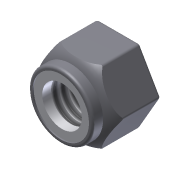
# Autodesk Inventor part: 10-32 regular lock nut
Saved by Autodesk Inventor 2011 (Build 150239000, 239)
## iProperties
Created: 2011-07-10
Part Number: 10-32 regular lock nut
Document SubType Name: Modeling
Designer: Dan Niemitalo
Density: 6.53812 g/cm^3
Material: Steel
Mass: 8.618 g
Surface Area: 11.454 cm^2
Volume: 1.31812 cm^3
Author: Dan Niemitalo
Autodesk Inventor part; units mm, degrees
ref_plane "YZ Plane" through (0, 0, 0) normal (1, 0, 0) x (0, 1, 0)
ref_plane "XZ Plane" through (0, 0, 0) normal (0, 1, 0) x (-1, 0, 0)
ref_plane "XY Plane" through (0, 0, 0) normal (0, 0, 1) x (1, 0, 0)
sketch "Sketch1" plane through (0, 0, 0) normal (0, 0, 1) x (1, 0, 0)
  line L0 (-4.1244, 7.1437) -> (4.1244, 7.1437)
  line L1 (4.1244, 7.1437) -> (8.2489, 0)
  line L2 (8.2489, 0) -> (4.1244, -7.1437)
  line L3 (4.1244, -7.1437) -> (-4.1244, -7.1437)
  line L4 (-4.1244, -7.1437) -> (-8.2489, 0)
  line L5 (-8.2489, 0) -> (-4.1244, 7.1437)
  point P0 (0, 0)
  point P1 (0, 0)
  dimension "d0" = 14.2875
  constraints: 12 end point, 1 coincident, 1 horizontal, 13 other
  measures "d0" distance between parallel lines of L3 L0
extrude "Extrusion1" add sketch "Sketch1" along normal blind 9.525
sketch "Sketch3" plane through (0, 0, 9.525) normal (0, 0, 1) x (1, 0, 0)
  circle A0 centre (0, 0) radius 6.35
  dimension "d3" = 12.7
  constraints: 1 centre point, 1 coincident
  measures "d3" diameter of A0
extrude "Extrusion2" add sketch "Sketch3" along normal blind 1.9844
sketch "Sketch8" plane through (0, 0, 11.5094) normal (0, 0, 1) x (1, 0, 0)
  circle A0 centre (0, 0) radius 6.35 projected
  circle A1 centre (0, 0) radius 5.5563
  circle A2 centre (0, 0) radius 5.1594
  dimension "d14" = 11.1125
  dimension "d28" = 10.3187
  constraints: 2 centre point, 2 coincident
  measures "d14" diameter of A1
  measures "d28" diameter of A2
extrude "Extrusion3" cut sketch "Sketch8" against normal blind 0.254 contours A1 | A2
sketch "Sketch9" plane through (0, 0, 0) normal (0, 0, -1) x (-1, 0, 0)
  point P0 (0, 0)
hole "Hole2" at (0, 0, 0) direction (0, 0, 1) diameter 7.7978 end through all thread size "3/8-16 UNC" class "2B" standard "ANSI Unified Screw Threads"
sketch "Sketch10" plane through (0, 0, 0) normal (0, 1, 0) x (-1, 0, 0)
  line L0 (-8.2489, 9.525) -> (-4.1244, 9.525) projected
  line L1 (-4.1244, 0) -> (-4.1244, 9.525) projected
  line L2 (-8.2489, 0) -> (-4.1244, 0) projected
  line L3 (-8.2489, 0) -> (-8.2489, 9.525) projected
  line L4 (0, 0) -> (0, 6.9243)
  arc A0 (-4.572, 9.525) -> (-8.2489, 7.3406) centre (-4.572, 5.3382) ccw
  line L5 (-8.2489, 7.3406) -> (-8.2489, 9.525)
  line L6 (-4.572, 9.525) -> (-8.2489, 9.525)
  dimension "d24" = 4.572
  constraints: 6 end point, 2 parallel, 2 point on circle, 2 point on line, 2 tangent, 1 centre point, 1 collinear
  measures "d24" distance from line of L4 L6.start
revolve "Revolution2" cut sketch "Sketch10" angle 360 about axis through (0, 0, 0) along (0, 0, 1) contours L0 A0 L3
fillet "Fillet1" radius 0.508 12 edges at (-4.1244, -7.1437, 3.6703) (4.1244, -7.1437, 3.6703) (8.2489, 0, 3.6703) (4.1244, 7.1437, 3.6703) (-8.2489, 0, 3.6703) (-4.1244, 7.1437, 3.6703) (0, 7.1437, 0) (6.1867, 3.5719, 0) (6.1867, -3.5719, 0) (0, -7.1437, 0) (-6.1867, -3.5719, 0) (-6.1867, 3.5719, 0)
fillet "Fillet2" radius 0.508 1 edges at (-6.35, 0, 11.5094)
body "Solid1"
